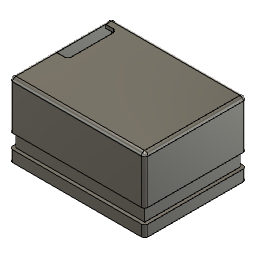
siren-controller-box v2 (Autodesk Fusion 360 design; units mm, degrees)
Autodesk Fusion 360 part; units mm, degrees
note: some values were not read from the file. Set by a fixed rule: which face or edge a step refers to.
sketch "Sketch1" plane through (0, 0, 0) normal (0, 1, 0) x (1, 0, 0)
  line L0 (-75, 25) -> (-14, 25)
  line L1 (-14, 25) -> (-14, -21)
  line L2 (-14, -21) -> (-75, -21)
  line L3 (-75, -21) -> (-75, 25)
  dimension "d5" = 61
  dimension "d6" = 46
  constraint horizontal L0
  constraint vertical L1
  constraint horizontal L2
  constraint vertical L3
  measures "d5" distance of L0.start L0.end
  measures "d6" distance of L0.start L2.end
extrude "Extrude1" add sketch "Sketch1" along normal blind 33 makes body 1
sketch "Sketch4" plane through (0, 0, 21) normal (0, 0, 1) x (1, 0, 0)
  line L0 (-75, 0) -> (-14, 0)
  line L1 (-14, 0) -> (-14, 33)
  line L2 (-14, 33) -> (-75, 33)
  line L3 (-75, 33) -> (-75, 0)
  line L4 (-75, 0) -> (-14, 0)
  line L5 (-14, 0) -> (-14, 11.5)
  line L6 (-14, 11.5) -> (-75, 11.5)
  line L7 (-75, 11.5) -> (-75, 0)
  dimension "d15" = 61
  dimension "d16" = 11.5
  constraint horizontal L4
  constraint vertical L5
  constraint horizontal L6
  constraint vertical L7
  constraint coincident L0.start L3.end
  measures "d15" distance of L0.start L0.end
  measures "d16" distance of L0.start L6.end
split "Split2" by curves path "Sketch4" along L4 L5 L6 L7 bodies 1 makes body 2 at (-54.6667, 33, -9.6667)
shell "Shell1" thickness 3 removed faces 1 at (-34.3333, 11.5, -9.6667) on bodies 1
shell "Shell2" thickness 1.5 removed faces 1 at (-34.3333, 11.5, -9.6667) on bodies 2
move_face "OffsetFaces1" offset -1.5 1 faces at (-53.6667, 3, -8.6667) on bodies 1
sketch "Sketch5" plane through (0, 0, 21) normal (0, 0, 1) x (1, 0, 0)
  line L0 (-14, 11.5) -> (-75, 11.5)
  line L1 (-75, 11.5) -> (-75, 0)
  line L2 (-75, 0) -> (-14, 0)
  line L3 (-14, 0) -> (-14, 11.5)
  line L4 (-75, 5) -> (-14, 5)
  point P0 (-75, 5)
  point P1 (-75, 5)
  point P2 (-75, 5)
  dimension "d20" = 5
  dimension "d21" = 61
  constraint coincident L1 P2
  constraint coincident P2 P1
  constraint perpendicular L3 L4
  measures "d20" distance of L1.end P2
  measures "d21" distance of P2 L4.end
sketch "Sketch6" plane through (-14, 0, 0) normal (1, 0, 0) x (0, 0, -1)
  line L0 (25, 11.5) -> (-21, 11.5)
  line L1 (-21, 11.5) -> (-21, 0)
  line L2 (-21, 0) -> (25, 0)
  line L3 (25, 0) -> (25, 11.5)
  line L4 (-21, 5) -> (25, 5)
  point P0 (-21, 5)
  dimension "d22" = 46
  constraint coincident P0 L4.start
  constraint perpendicular L3 L4
  measures "d22" distance of P0 L4.end
sketch "Sketch7" plane through (0, 0, -25) normal (0, 0, -1) x (-1, 0, 0)
  line L0 (75, 11.5) -> (14, 11.5)
  line L1 (14, 11.5) -> (14, 0)
  line L2 (14, 0) -> (75, 0)
  line L3 (75, 0) -> (75, 11.5)
  line L4 (14, 5) -> (75, 5)
  point P0 (14, 5)
  dimension "d23" = 61
  constraint coincident P0 L4.start
  constraint perpendicular L1 L4
  measures "d23" distance of P0 L4.end
sketch "Sketch8" plane through (-75, 0, 0) normal (-1, 0, 0) x (0, 0, 1)
  line L0 (21, 11.5) -> (-25, 11.5)
  line L1 (-25, 11.5) -> (-25, 0)
  line L2 (-25, 0) -> (21, 0)
  line L3 (21, 0) -> (21, 11.5)
  line L4 (-25, 5) -> (21, 5)
  point P0 (-25, 5)
  point P1 (21, 5)
  constraint coincident P0 L4.start
  constraint coincident P1 L4.end
extrude "Extrude2" cut sketch "Sketch8" against normal blind 1.5 contours L0 L1 L3 L4 bodies 1
extrude "Extrude3" cut sketch "Sketch7" against normal blind 1.5 contours L0 L1 L3 L4 bodies 1
extrude "Extrude4" cut sketch "Sketch6" against normal blind 1.5 contours L0 L1 L3 L4 bodies 1
extrude "Extrude5" cut sketch "Sketch5" against normal blind 1.5 contours L0 L1 L3 L4 bodies 1
fillet "Fillet4" radius 1.5 12 edges at (-14, 2.5, 21) (-14, 2.5, -25) (-75, 2.5, 21) (-75, 2.5, -25) (-14, 22.25, 21) (-14, 33, -2) (-44.5, 33, 21) (-75, 33, -2) (-44.5, 33, -25) (-14, 22.25, -25) (-75, 22.25, 21) (-75, 22.25, -25) on bodies 1 2
sketch "Sketch10" plane through (-73.5, 0, 0) normal (-1, 0, 0) x (0, 0, 1)
  line L0 (19.5, 5) -> (19.5, 11.5)
  line L1 (19.5, 11.5) -> (-23.5, 11.5)
  line L2 (-23.5, 11.5) -> (-23.5, 5)
  line L3 (-23.5, 5) -> (19.5, 5)
  line L4 (-20.5, 8) -> (1.5, 8)
  line L5 (1.5, 8) -> (1.5, 11.5)
  line L6 (1.5, 11.5) -> (-20.5, 11.5)
  line L7 (-20.5, 11.5) -> (-20.5, 8)
  point P0 (-20.5, 8)
  dimension "d34" = 3
  dimension "d35" = 3
  dimension "d36" = 22
  constraint horizontal L4
  constraint vertical L5
  constraint horizontal L6
  constraint vertical L7
  constraint coincident P0 L4.start
  measures "d34" distance of L2 P0
  measures "d35" distance of L3 P0
  measures "d36" distance of P0 L4.end
extrude "Extrude6" cut sketch "Sketch10" against normal blind 12 contours L1 L4 L5 L6 L7 bodies 1
sketch "Sketch11" plane through (-75, 0, 0) normal (-1, 0, 0) x (0, 0, 1)
  line L0 (-23.5, 31.5) -> (-23.5, 11.5)
  line L1 (-23.5, 11.5) -> (19.5, 11.5)
  line L2 (19.5, 11.5) -> (19.5, 31.5)
  line L3 (19.5, 31.5) -> (-23.5, 31.5)
  line L4 (-20.511, 11.5) -> (1.489, 11.5)
  line L5 (1.489, 11.5) -> (1.489, 24.5)
  line L6 (1.489, 24.5) -> (-20.511, 24.5)
  line L7 (-20.511, 24.5) -> (-20.511, 11.5)
  point P0 (-20.5, 11.9)
  dimension "d39" = 22
  dimension "d40" = 13
  constraint horizontal L4
  constraint vertical L5
  constraint horizontal L6
  constraint vertical L7
  constraint coincident L1 L4.start
  measures "d39" distance of L4.start L4.end
  measures "d40" distance of L4.start L6.end
extrude "Extrude7" cut sketch "Sketch11" against normal blind 25 contours L1 L4 L5 L6 L7 bodies 2
sketch "Sketch12" plane through (0, 33, 0) normal (0, 1, 0) x (-1, 0, 0)
  line L0 (15.5, -23.5) -> (73.5, -23.5)
  line L1 (73.5, -23.5) -> (73.5, 19.5)
  line L2 (73.5, 19.5) -> (15.5, 19.5)
  line L3 (15.5, 19.5) -> (15.5, -23.5)
  line L4 (73.5, -20.9215) -> (68.5, -20.9215)
  line L5 (68.5, -20.9215) -> (68.5, 1.0785)
  line L6 (68.5, 1.0785) -> (73.5, 1.0785)
  line L7 (73.5, 1.0785) -> (73.5, -20.9215)
  dimension "d43" = 5
  dimension "d44" = 22
  constraint horizontal L4
  constraint vertical L5
  constraint horizontal L6
  constraint vertical L7
  constraint coincident L1 L4.start
  measures "d43" distance of L4.start L4.end
  measures "d44" distance of L4.start L6.end
extrude "Extrude8" cut sketch "Sketch12" against normal blind 11 contours L1 L4 L5 L6 L7 bodies 2
fillet "Fillet5" radius 1.5 2 edges at (-68.5, 32.25, -20.9215) (-68.5, 32.25, 1.0785) on bodies 2
equation "length = 55 mm"
equation "width = 40 mm"
equation "height = 25 mm"
equation "thickness = 1.5 mm"
equation "d5 = length + 4 * thickness"
equation "d6 = width + 4 * thickness"
equation "overhang = 5 mm"
equation "d8 = height + overhang + 2 * thickness"
equation "d15 = length + 4 * thickness"
equation "d16 = thickness + 2 * overhang"
equation "d17 = 2 * thickness"
equation "d18 = thickness"
equation "d19 = -thickness"
equation "d20 = overhang"
equation "d21 = length + 4 * thickness"
equation "d22 = width + 4 * thickness"
equation "d23 = length + 4 * thickness"
equation "d24 = -thickness"
equation "d26 = -thickness"
equation "d28 = -thickness"
equation "d30 = -thickness"
equation "d33 = thickness"
equation "d47 = thickness"
named bodies: "Bottom", "top"
